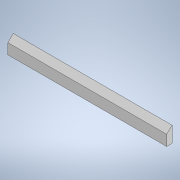
# Autodesk Inventor part: ball_ramp
Saved by Autodesk Inventor 2020 (Build 240168000, 168)
## iProperties
Created: 2021-03-06
Part Number: ball_ramp
Material: Generic
Document SubType Name: Modeling
Designer: Harry
Density: 1 g/cm^3
Appearance: Default
Author: Harry
Autodesk Inventor part; units mm, degrees
ref_plane "YZ Plane" through (0, 0, 0) normal (1, 0, 0) x (0, 1, 0)
ref_plane "XZ Plane" through (0, 0, 0) normal (0, 1, 0) x (-1, 0, 0)
ref_plane "XY Plane" through (0, 0, 0) normal (0, 0, 1) x (1, 0, 0)
sketch "Sketch1" plane through (0, 0, 0) normal (0, 0, 1) x (1, 0, 0)
  line L0 (150, -15) -> (-150, -15)
  line L1 (-150, -15) -> (-150, 15)
  line L2 (-150, 15) -> (150, 15)
  line L3 (150, 15) -> (150, -15)
  line L4 (150, -15) -> (-150, 15) construction
  line L5 (-150, -15) -> (150, 15) construction
  point P0 (0, 0)
  dimension "d0" = 300
  dimension "d1" = 30
  constraints: 12 end point, 2 midpoint, 2 parallel, 1 horizontal, 1 perpendicular
  measures "d0" distance of L1.end L2.end
  measures "d1" distance of L0.end L1.end
extrude "Extrusion1" add sketch "Sketch1" along normal blind 10
chamfer "Chamfer1" distance 10 angle 45 1 edges at (0, 15, 10)
body "Solid1"
